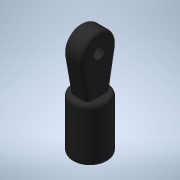
# Autodesk Inventor part: wheel_shock_end
Saved by Autodesk Inventor 2020 (Build 240168000, 168)
## iProperties
Created: 2016-01-05
Part Number: wheel_shock_end
Material: Genérico
Document SubType Name: Modeling
Designer: MIGUEL ANGEL
Density: 1 g/cm^3
Appearance: Goma - Negro
Author: MIGUEL ANGEL
Autodesk Inventor part; units mm, degrees
ref_plane "YZ Plane" through (0, 0, 0) normal (1, 0, 0) x (0, 1, 0)
ref_plane "XZ Plane" through (0, 0, 0) normal (0, 1, 0) x (-1, 0, 0)
ref_plane "XY Plane" through (0, 0, 0) normal (0, 0, 1) x (1, 0, 0)
sketch "Boceto1" plane through (0, 0, 0) normal (0, 0, 1) x (1, 0, 0)
  circle A0 centre (0, 0) radius 10
  dimension "d0" = 20
  constraints: 1 centre point, 1 coincident
  measures "d0" diameter of A0
extrude "Extrusión1" add sketch "Boceto1" along normal blind 30
sketch "Boceto2" plane through (0, 0, 0) normal (1, 0, 0) x (0, 1, 0)
  line L0 (10, 30) -> (-10, 30) projected
  line L1 (-10, 0) -> (10, 0) projected
  line L2 (10, 30) -> (-10, 30) projected
  line L3 (6.3751, 30) -> (9.8481, 49.6962)
  arc A0 (9.8481, 49.6962) -> (0, 61.4326) centre (0, 51.4326) ccw
  line L4 (0, 73.9906) -> (0, 23.9809)
  line L5 (-6.3751, 30) -> (-9.8481, 49.6962)
  arc A1 (0, 61.4326) -> (-9.8481, 49.6962) centre (0, 51.4326) ccw
  line L6 (6.3751, 30) -> (-6.3751, 30)
  point P0 (0, 0)
  point P1 (0, 30)
  dimension "d3" = 10
  dimension "d4" = 20
  dimension "d5" = 100
  constraints: 8 end point, 4 point on circle, 2 centre point, 2 symmetric about line, 2 vertical alignment, 1 collinear, 1 midpoint, 1 point on line, 1 tangent, 1 vertical, 1 other
  measures "d3" radius of A0
  measures "d4" distance of L3.start L3.end
  measures "d5" angle of L0 L3
extrude "Extrusión2" add sketch "Boceto2" along normal mid plane 10.5
hole "Agujero1" at (5.25, 0, 51.4326) direction (-1, 0, 0) diameter 6 end through all
hole "Agujero2" at (0, 0, 0) direction (0, 0, 1) diameter 6 depth 26 tip angle 118
fillet "Empalme1" radius 2 8 edges at (5.25, -8.1116, 39.8481) (5.25, 8.1116, 39.8481) (5.25, -7.6604, 57.8605) (-5.25, 8.1116, 39.8481) (-5.25, -8.1116, 39.8481) (-5.25, 7.6604, 57.8605) (-10, 0, 30) (-10, 0, 0)
